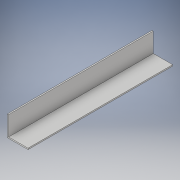
# Autodesk Inventor part: Hook7in L Channel
Saved by Autodesk Inventor 2018 (Build 220112000, 112)
## iProperties
Created: 2020-01-24
Part Number: Hook7in L Channel
Material: Generic
Document SubType Name: Modeling
Designer: s-2513398
Density: 1 g/cm^3
Appearance: Default
Author: s-2513398
Autodesk Inventor part; units mm, degrees
ref_plane "YZ Plane" through (0, 0, 0) normal (1, 0, 0) x (0, 1, 0)
ref_plane "XZ Plane" through (0, 0, 0) normal (0, 1, 0) x (-1, 0, 0)
ref_plane "XY Plane" through (0, 0, 0) normal (0, 0, 1) x (1, 0, 0)
sketch "Sketch1" plane through (0, 0, 0) normal (0, 0, 1) x (1, 0, 0)
  line L0 (0, 0) -> (25.4, 0)
  line L1 (0, 25.4053) -> (0, 0)
  line L2 (1.5875, 22.2862) -> (1.5875, 23.8178) construction
  line L3 (1.5875, 25.4053) -> (1.5875, 1.5875)
  line L4 (1.5875, 1.5875) -> (25.4, 1.5875)
  line L5 (0, 25.4053) -> (1.5875, 25.4053)
  line L6 (25.4, 1.5875) -> (25.4, 0)
  constraints: 14 end point, 2 horizontal, 1 perpendicular, 1 vertical
extrude "Extrusion2" add sketch "Sketch1" along normal blind 177.8
body "Solid2"
